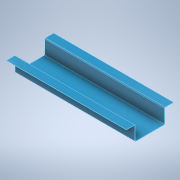
# Autodesk Inventor part: Cubby Sheet Metal
Saved by Autodesk Inventor 2021 (Build 250183000, 183)
## iProperties
Created: 2021-02-13
Part Number: Cubby Sheet Metal
Material: Steel, Mild
Document SubType Name: Sheet Metal
Designer: bl17
Density: 7.85 g/cm^3
Sheet Metal Rule: Default
Appearance: Sky Blue Dark
Author: bl17
Autodesk Inventor part; units mm, degrees
ref_plane "YZ Plane" through (0, 0, 0) normal (1, 0, 0) x (0, 1, 0)
ref_plane "XZ Plane" through (0, 0, 0) normal (0, 1, 0) x (-1, 0, 0)
ref_plane "XY Plane" through (0, 0, 0) normal (0, 0, 1) x (1, 0, 0)
sketch "Sketch1" plane through (0, 0, 0) normal (0, 1, 0) x (-1, 0, 0)
  line L0 (254, 63.5) -> (-254, 63.5)
  line L1 (-254, 63.5) -> (-254, -63.5)
  line L2 (-254, -63.5) -> (254, -63.5)
  line L3 (254, -63.5) -> (254, 63.5)
  line L4 (254, 63.5) -> (-254, -63.5) construction
  line L5 (-254, 63.5) -> (254, -63.5) construction
  point P0 (0, 0)
  dimension "d0" = 508
  dimension "d1" = 127
  constraints: 12 end point, 2 midpoint, 2 parallel, 1 horizontal, 1 perpendicular
  measures "d0" distance of L2.end L1.end
  measures "d1" distance of L1.end L0.end
extrude "Extrusion1" add sketch "Sketch1" along normal blind 1.5875
sketch "Sketch2" plane through (254, 0, 61.9125) normal (0, 0, 1) x (1, 0, 0)
  line L0 (-508, 0) -> (0, 0)
  line L1 (0, 0) -> (0, 63.5)
  line L2 (0, 63.5) -> (-508, 63.5)
  line L3 (-508, 63.5) -> (-508, 0)
  constraints: 6 end point, 1 horizontal, 1 perpendicular, 1 vertical
edge flange "Flange1" height 63.5 angle 90 thickness 1.5875 bend radius 1.5875 thickness toward (0, 0, 1) relief straight relief width 1.5875 relief depth 0.7937 edges at (0, 1.5875, 63.5) wall of the first edge with corners at (-254, 0, 61.9125) (254, 0, 61.9125) (254, 63.5, 61.9125) (-254, 63.5, 61.9125)
bend "Bend1"
corner "Corner1"
sketch "Sketch3" plane through (-254, 61.9125, 61.9125) normal (0, 1, 0) x (-1, 0, 0)
  line L0 (-508, 0) -> (0, 0)
  line L1 (0, 0) -> (0, 38.1)
  line L2 (0, 38.1) -> (-508, 38.1)
  line L3 (-508, 38.1) -> (-508, 0)
  constraints: 6 end point, 1 horizontal, 1 perpendicular, 1 vertical
edge flange "Flange2" height 38.1 angle 90 thickness 1.5875 bend radius 1.5875 thickness toward (0, 1, 0) relief straight relief width 1.5875 relief depth 0.7937 edges at (0, 63.5, 63.5) wall of the first edge with corners at (254, 61.9125, 61.9125) (-254, 61.9125, 61.9125) (-254, 61.9125, 100.0125) (254, 61.9125, 100.0125)
bend "Bend2"
corner "Corner2"
sketch "Sketch4" plane through (-254, 0, -61.9125) normal (0, 0, -1) x (-1, 0, 0)
  line L0 (-508, 0) -> (0, 0)
  line L1 (0, 0) -> (0, 63.5)
  line L2 (0, 63.5) -> (-508, 63.5)
  line L3 (-508, 63.5) -> (-508, 0)
  constraints: 6 end point, 1 horizontal, 1 perpendicular, 1 vertical
edge flange "Flange3" height 63.5 angle 90 thickness 1.5875 bend radius 1.5875 thickness toward (0, 0, -1) relief straight relief width 1.5875 relief depth 0.7937 edges at (0, 1.5875, -63.5) wall of the first edge with corners at (254, 0, -61.9125) (-254, 0, -61.9125) (-254, 63.5, -61.9125) (254, 63.5, -61.9125)
bend "Bend3"
corner "Corner3"
sketch "Sketch5" plane through (254, 61.9125, -61.9125) normal (0, 1, 0) x (-1, 0, 0)
  line L0 (508, 0) -> (0, 0)
  line L1 (0, 0) -> (0, -38.1)
  line L2 (0, -38.1) -> (508, -38.1)
  line L3 (508, -38.1) -> (508, 0)
  constraints: 6 end point, 1 horizontal, 1 perpendicular, 1 vertical
edge flange "Flange4" height 38.1 angle 90 thickness 1.5875 bend radius 1.5875 thickness toward (0, 1, 0) relief straight relief width 1.5875 relief depth 0.7937 edges at (0, 63.5, -63.5) wall of the first edge with corners at (-254, 61.9125, -61.9125) (254, 61.9125, -61.9125) (254, 61.9125, -100.0125) (-254, 61.9125, -100.0125)
bend "Bend4"
corner "Corner4"
equation "\"d4\" = Thickness"
equation "\"d5\" = BendReliefWidth"
equation "\"d6\" = BendReliefDepth"
equation "\"d7\" = MinimumRemnant"
equation "\"d8\" = TransitionRadius"
equation "\"d11\" = BendRadius"
equation "\"d12\" = CornerReliefSize"
equation "\"d13\" = GapSize"
equation "\"d14\" = JacobiRadiusSize"
equation "\"d15\" = BendReliefWidth"
equation "\"d16\" = BendReliefDepth"
equation "\"d17\" = MinimumRemnant"
equation "\"d18\" = TransitionRadius"
equation "\"d21\" = BendRadius"
equation "\"d22\" = CornerReliefSize"
equation "\"d23\" = GapSize"
equation "\"d24\" = JacobiRadiusSize"
equation "\"d25\" = BendReliefWidth"
equation "\"d26\" = BendReliefDepth"
equation "\"d27\" = MinimumRemnant"
equation "\"d28\" = TransitionRadius"
equation "\"d31\" = BendRadius"
equation "\"d32\" = CornerReliefSize"
equation "\"d33\" = GapSize"
equation "\"d34\" = JacobiRadiusSize"
equation "\"d35\" = BendReliefWidth"
equation "\"d36\" = BendReliefDepth"
equation "\"d37\" = MinimumRemnant"
equation "\"d38\" = TransitionRadius"
equation "\"d41\" = BendRadius"
equation "\"d42\" = CornerReliefSize"
equation "\"d43\" = GapSize"
equation "\"d44\" = JacobiRadiusSize"
equation "\"BendRadius\" = Thickness"
equation "\"BendReliefWidth\" = Thickness"
equation "\"BendReliefDepth\" = 0.5 * Thickness"
equation "\"CornerReliefSize\" = 4 * Thickness"
equation "\"MinimumRemnant\" = 2 * Thickness"
equation "\"TransitionRadius\" = BendRadius"
equation "\"JacobiRadiusSize\" = Thickness"
equation "\"GapSize\" = Thickness"
equation "\"Thickness\" = 1.5875"
body "Solid1"
